# Autodesk Inventor part: TSOP57238TT1
Saved by Autodesk Inventor 2016 SP1 (Build 200210100, 210)
## iProperties
Created: 2015-11-19
Part Number: TSOP57238TT1
Material: Generic
Document SubType Name: Modeling
Designer: PhillipD
Density: 1 g/cm^3
Appearance: TSOP572, TSOP57238TT1
Author: PhillipD
Autodesk Inventor part; units mm, degrees
ref_plane "YZ Plane" through (0, 0, 0) normal (1, 0, 0) x (0, 1, 0)
ref_plane "XZ Plane" through (0, 0, 0) normal (0, 1, 0) x (-1, 0, 0)
ref_plane "XY Plane" through (0, 0, 0) normal (0, 0, 1) x (1, 0, 0)
sketch "TSOP572, TSOP57238TT1_78" plane through (0, 0, 0) normal (0, 0, 1) x (1, 0, 0)
  line L0 (-2.8016, 2.0385) -> (2.0385, 2.0385)
  line L1 (2.0385, 2.0385) -> (2.0385, -2.0016)
  line L2 (2.0385, -2.0016) -> (-2.8016, -2.0016)
  line L3 (-2.8016, -2.0016) -> (-2.8016, 2.0385)
  constraints: 8 end point
extrude "Extrusion1" add sketch "TSOP572, TSOP57238TT1_78" along normal blind 1
body "Solid1"
